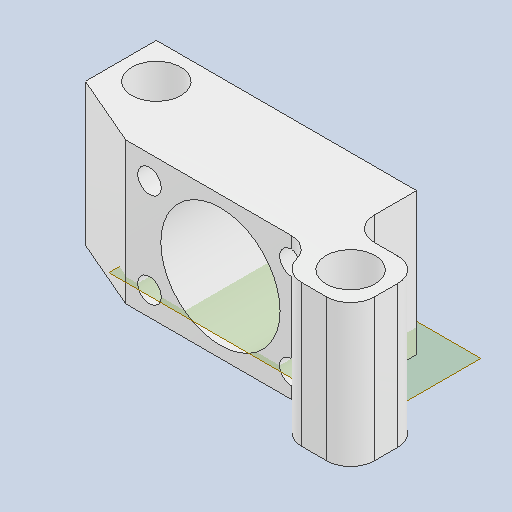
# Autodesk Inventor part: Motor Sleeve
Saved by Autodesk Inventor 2023.2 (Build 272271000, 271)
## iProperties
Created: 2023-04-12
Part Number: Motor Sleeve
Material: UHMW, White
Document SubType Name: Modeling
Designer: Nathan Cai
Density: 0.94 g/cm^3
Appearance: Smooth - White
Mass: 5.55755 g
Surface Area: 47.1476 cm^2
Volume: 5.91229 cm^3
Author: Nathan Cai
Autodesk Inventor part; units mm, degrees
ref_plane "YZ Plane" through (0, 0, 0) normal (1, 0, 0) x (0, 1, 0)
ref_plane "XZ Plane" through (0, 0, 0) normal (0, 1, 0) x (-1, 0, 0)
ref_plane "XY Plane" through (0, 0, 0) normal (0, 0, 1) x (1, 0, 0)
sketch "Sketch1" plane through (0, 0, 0) normal (0, 0, 1) x (1, 0, 0)
  line L0 (-9.525, -6.35) -> (9.525, -6.35) construction
  line L1 (9.525, -6.35) -> (9.525, 6.35) construction
  line L2 (9.525, 6.35) -> (-9.525, 6.35) construction
  line L3 (-9.525, 6.35) -> (-9.525, -6.35) construction
  line L4 (-9.525, -6.35) -> (9.525, 6.35) construction
  line L5 (9.525, -6.35) -> (-9.525, 6.35) construction
  circle A0 centre (0, 0) radius 8
  circle A1 centre (-9.525, 6.35) radius 1.5875
  circle A2 centre (9.525, 6.35) radius 1.5875
  circle A3 centre (-9.525, -6.35) radius 1.5875
  circle A4 centre (9.525, -6.35) radius 1.5875
  line L6 (-12.7, -9.525) -> (12.7, -9.525)
  line L7 (12.7, -9.525) -> (12.7, 9.525)
  line L8 (12.7, 9.525) -> (-12.7, 9.525)
  line L9 (-12.7, 9.525) -> (-12.7, -9.525)
  line L10 (-12.7, -9.525) -> (12.7, 9.525) construction
  line L11 (12.7, -9.525) -> (-12.7, 9.525) construction
  dimension "d0" = 19.05
  dimension "d1" = 12.7
  dimension "d2" = 16
  dimension "d3" = 3.175
  dimension "d6" = 19.05
  dimension "d9" = 12.7
  dimension "d12" = 25.4
  dimension "d13" = 19.05
  constraints: 24 end point, 5 centre point, 4 midpoint, 4 parallel, 3 horizontal, 2 coincident, 2 perpendicular, 1 vertical, 6 other
  measures "d0" distance of L2.end L1.end
  measures "d1" distance of L1.end L0.end
  measures "d2" diameter of A0
  measures "d3" diameter of A1
  measures "d6" distance of A1.centre A2.centre
  measures "d9" distance of A1.centre A3.centre
  measures "d12" distance of L8.end L7.end
  measures "d13" distance of L7.end L6.end
extrude "Extrusion1" add sketch "Sketch1" along normal blind 13.625
ref_plane "Work Plane1" through (-12.7, -6.35, 0) normal (0, -1, 0) x (1, 0, 0)
sketch "Sketch2" plane through (-12.7, -9.525, 0) normal (0, -1, 0) x (1, 0, 0)
  line L0 (25.4, 0) -> (25.4, 13.625) projected
  line L1 (25.4, 0) -> (34.925, 0)
  line L2 (34.925, 0) -> (34.925, 9.525)
  line L3 (34.925, 9.525) -> (25.4, 9.525) construction
  line L4 (25.4, 9.525) -> (25.4, 0)
  line L5 (12.7, 0) -> (12.7, 13.625) construction
  line L6 (4.7, 13.625) -> (20.7, 13.625) projected
  line L7 (34.925, 9.525) -> (25.4, 0) construction
  circle A0 centre (30.1625, 4.7625) radius 3.302 construction
  line L8 (0, 0) -> (0, 13.625)
  line L9 (0, 0) -> (-9.525, 0)
  line L10 (-9.525, 0) -> (-9.525, 9.525)
  line L11 (-9.525, 9.525) -> (0, 9.525)
  line L12 (0, 9.525) -> (0, 0)
  line L13 (-9.525, 9.525) -> (0, 0) construction
  circle A1 centre (-4.7625, 4.7625) radius 3.302
  circle A2 centre (30.1625, 13.625) radius 3.302
  line L14 (25.4, 13.625) -> (0, 13.625) projected
  line L15 (30.1625, 4.7625) -> (30.1625, 13.625) construction
  line L16 (25.4, 18.3875) -> (34.925, 18.3875)
  line L17 (34.925, 18.3875) -> (34.925, 8.8625)
  line L18 (34.925, 8.8625) -> (25.4, 8.8625)
  line L19 (25.4, 8.8625) -> (25.4, 18.3875)
  line L20 (25.4, 18.3875) -> (34.925, 8.8625) construction
  line L21 (34.925, 18.3875) -> (25.4, 8.8625) construction
  point P0 (25.4, 9.525)
  dimension "d16" = 9.525
  dimension "d17" = 9.525
  dimension "d18" = 6.604
  dimension "d29" = 6.604
  dimension "d30" = 9.525
  dimension "d31" = 9.525
  constraints: 38 end point, 6 symmetric about line, 4 midpoint, 4 parallel, 3 centre point, 2 horizontal, 2 perpendicular, 1 point on line, 1 vertical, 1 other
  measures "d16" distance of L3.end L2.end
  measures "d17" distance of L2.end L1.end
  measures "d18" diameter of A0
  measures "d29" diameter of A2
  measures "d30" distance of L17.end L18.end
  measures "d31" distance of L16.end L17.end
extrude "Extrusion2" add sketch "Sketch2" against normal blind 19.05 contours L0 L19 L16 L17 L2 L18 | L9 L10 L11 L8
chamfer "Chamfer2" distance 4.1 distance2 9.525 1 edges at (-12.7, 0, 9.525) measured on face at (-12.7, 0, 10.025)
fillet "Fillet2" radius 3.175 5 edges at (12.7, 0, 13.625) (12.7, 0, 18.3875) (22.225, 0, 18.3875) (22.225, 0, 8.8625) (12.7, 0, 8.8625)
equation "\"d6\" = d0"
equation "\"d9\" = d1"
body "Solid1"
